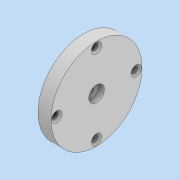
# Autodesk Inventor part: 외부 바퀴 서포터
Saved by Autodesk Inventor 2020 (Build 240168000, 168)
## iProperties
Created: 2020-05-04
Part Number: 외부 바퀴 서포터
Material: 일반
Document SubType Name: Modeling
Designer: sbahn
Density: 1 g/cm^3
Appearance: 기본값
Author: sbahn
Autodesk Inventor part; units mm, degrees
ref_plane "YZ Plane" through (0, 0, 0) normal (1, 0, 0) x (0, 1, 0)
ref_plane "XZ Plane" through (0, 0, 0) normal (0, 1, 0) x (-1, 0, 0)
ref_plane "XY Plane" through (0, 0, 0) normal (0, 0, 1) x (1, 0, 0)
sketch "스케치1" plane through (0, 0, 0) normal (1, 0, 0) x (0, 1, 0)
  circle A0 centre (0, 0) radius 17.5
  circle A1 centre (0, 0) radius 1
  dimension "d0" = 35
  dimension "d1" = 2
  constraints: 2 centre point, 2 coincident
  measures "d0" diameter of A0
  measures "d1" diameter of A1
extrude "돌출1" add sketch "스케치1" along normal blind 5
sketch "스케치2" plane through (5, 0, 0) normal (1, 0, 0) x (0, 0, -1)
  circle A0 centre (0, 0) radius 3
  dimension "d4" = 6
  constraints: 1 centre point, 1 coincident
  measures "d4" diameter of A0
extrude "돌출2" cut sketch "스케치2" against normal blind 2
sketch "스케치3" plane through (5, 0, 0) normal (1, 0, 0) x (0, 0, -1)
  circle A0 centre (0, 0) radius 15.25
  line L0 (0, 0) -> (0, -17.6293)
  point P0 (0, -15.25)
  dimension "d7" = 30.5
  constraints: 2 end point, 1 coincident, 1 point on line, 1 vertical, 1 vertical alignment, 2 other
hole "구멍1" at (5, -15.25, 0) direction (-1, 0, 0) diameter 2.5 depth 10 tip angle 118 countersink diameter 4 countersink angle 90
pattern_circular "원형 패턴1" count 4 over 360 about axis through (0, 0, 0) along (1, 0, 0) of "구멍1"
